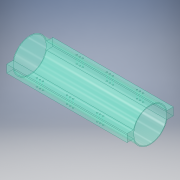
# Autodesk Inventor part: body
Saved by Autodesk Inventor 2019 (Build 230136000, 136)
## iProperties
Created: 2020-07-18
Part Number: body
Material: Generic
Document SubType Name: Modeling
Designer: Agus Prayudi
Density: 1 g/cm^3
Appearance: Indoor Pool
Author: Agus Prayudi
Autodesk Inventor part; units mm, degrees
ref_plane "YZ Plane" through (0, 0, 0) normal (1, 0, 0) x (0, 1, 0)
ref_plane "XZ Plane" through (0, 0, 0) normal (0, 1, 0) x (-1, 0, 0)
sketch "Sketch1" plane through (0, 0, 0) normal (1, 0, 0) x (0, 1, 0)
  circle A0 centre (0, 0) radius 54.5
  circle A1 centre (0, 0) radius 57
  dimension "d0" = 109
  dimension "d1" = 114
  constraints: 2 centre point, 2 coincident
  measures "d0" diameter of A0
  measures "d1" diameter of A1
extrude "Extrusion1" add sketch "Sketch1" along normal blind 400
sketch "Sketch2" plane through (400, 0, 0) normal (1, 0, 0) x (0, 0, -1)
  circle A0 centre (0, 0) radius 57 projected
  line L0 (-77, 0) -> (-77, 13)
  line L1 (-77, 13) -> (-77, -13)
  line L2 (-77, -13) -> (-55.4977, -13)
  line L3 (-77, 13) -> (-55.4977, 13)
  line L4 (-55.4977, 13) -> (-77, 13)
  line L5 (-77, 13) -> (-77, -13)
  line L6 (-77, -13) -> (-55.4977, -13)
  arc A1 (-55.4977, 13) -> (-55.4977, -13) centre (0, 0) ccw
  dimension "d5" = 13
  dimension "d6" = 26
  constraints: 14 end point, 3 collinear, 2 point on circle, 1 centre point, 1 perpendicular, 1 point on line, 3 other
  measures "d5" distance of L0.start L0.end
  measures "d6" distance of L0.end L1.end
extrude "Extrusion2" add sketch "Sketch2" against normal blind 400 contours A0 L2 L1 L0 L3
ref_plane "Work Plane1" through (0, 0, 0) normal (0, 0, 1) x (1, 0, 0)
mirror "Mirror1" about plane through (0, 0, 0) normal (0, 0, 1) of "Extrusion2"
sketch "Sketch3" plane through (400, 13, 77) normal (0, 1, 0) x (1, 0, 0)
  line L0 (-400, 21.5023) -> (-400, 0) projected
  line L1 (0, 0) -> (0, 21.5023) projected
  circle A0 centre (-200, 10.7511) radius 2.5
  circle A1 centre (-100, 10.7511) radius 2.5
  circle A2 centre (-300, 10.7511) radius 2.5
  circle A3 centre (-190, 10.7511) radius 2.5
  circle A4 centre (-210, 10.7511) radius 2.5
  circle A5 centre (-290, 10.7511) radius 2.5
  circle A6 centre (-310, 10.7511) radius 2.5
  circle A7 centre (-90, 10.7511) radius 2.5
  circle A8 centre (-110, 10.7511) radius 2.5
  point P0 (-400, 77)
  constraints: 9 centre point
extrude "Extrusion4" cut sketch "Sketch3" against normal blind 400
mirror "Mirror3" about plane through (0, 0, 0) normal (0, 0, 1) of "Extrusion4"
body "Solid1"
